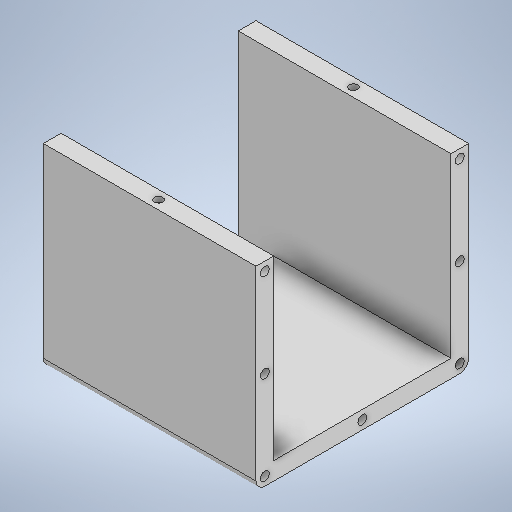
# Autodesk Inventor part: Fuselage_Body_Piece
Saved by Autodesk Inventor 2025.1 (Build 291241020, 241B)
## iProperties
Created: 2025-02-15
Part Number: Fuselage_Body_Piece
Material: Generic
Document SubType Name: Modeling
Designer: smyth
Density: 1 g/cm^3
Appearance: Default
Author: smyth
Autodesk Inventor part; units mm, degrees
ref_plane "YZ Plane" through (0, 0, 0) normal (1, 0, 0) x (0, 1, 0)
ref_plane "XZ Plane" through (0, 0, 0) normal (0, 1, 0) x (-1, 0, 0)
ref_plane "XY Plane" through (0, 0, 0) normal (0, 0, 1) x (1, 0, 0)
sketch "Sketch1" plane through (0, 0, 0) normal (0, 1, 0) x (-1, 0, 0)
  point P0 (0, 0)
sketch "Sketch2" plane through (0, 0, 0) normal (0, 1, 0) x (-1, 0, 0)
  line L0 (-76.2, 76.2) -> (76.2, 76.2)
  line L1 (76.2, 76.2) -> (76.2, -76.2)
  line L2 (76.2, -76.2) -> (-76.2, -76.2)
  line L3 (-76.2, -76.2) -> (-76.2, 76.2)
  line L4 (-76.2, 76.2) -> (76.2, -76.2) construction
  line L5 (76.2, 76.2) -> (-76.2, -76.2) construction
  point P0 (0, 0)
  dimension "d0" = 152.4
  dimension "d1" = 152.4
  constraints: 12 end point, 2 midpoint, 2 parallel, 1 horizontal, 1 perpendicular
  measures "d0" distance of L1.end L2.end
  measures "d1" distance of L0.end L1.end
extrude "Extrusion1" add sketch "Sketch2" along normal blind 12.7
sketch "Sketch3" plane through (0, 12.7, 0) normal (0, 1, 0) x (1, 0, 0)
  line L0 (76.2, 76.2) -> (-76.2, 76.2) projected
  line L1 (76.2, -76.2) -> (76.2, 76.2) projected
  line L2 (-76.2, 76.2) -> (76.2, 76.2)
  line L3 (76.2, 76.2) -> (76.2, 63.5)
  line L4 (76.2, 63.5) -> (-76.2, 63.5)
  line L5 (-76.2, 63.5) -> (-76.2, 76.2)
  line L6 (-76.2, -76.2) -> (76.2, -76.2)
  line L7 (76.2, -76.2) -> (76.2, -63.5)
  line L8 (76.2, -63.5) -> (-76.2, -63.5)
  line L9 (-76.2, -63.5) -> (-76.2, -76.2)
  point P0 (0, 0)
  point P1 (76.2, -76.2)
  dimension "d4" = 12.7
  dimension "d5" = 12.7
  dimension "d15" = 152.4
  constraints: 16 end point, 4 parallel, 2 horizontal, 2 perpendicular, 2 point on line
  measures "d4" distance between parallel lines of L4 L0
  measures "d5" distance between parallel lines of L8 L6
  measures "d15" distance of L6.start L6.end
extrude "Extrusion2" add sketch "Sketch3" along normal blind 127
fillet "Fillet1" radius 6.35 2 edges at (0, 0, 76.2) (0, 0, -76.2)
sketch "Sketch4" plane through (76.2, 12.7, -63.5) normal (1, 0, 0) x (0, 0, -1)
  circle A0 centre (-133.35, 120.65) radius 3.175
  circle A1 centre (-133.35, -6.35) radius 3.175
  circle A2 centre (-133.35, 57.15) radius 3.175
  circle A3 centre (6.35, 120.65) radius 3.175
  circle A4 centre (6.35, -6.35) radius 3.175
  circle A5 centre (6.35, 57.15) radius 3.175
  circle A6 centre (-63.5, -6.35) radius 3.175
  point P0 (-63.5, -12.7)
  dimension "d9" = 127
  constraints: 7 centre point
  measures "d9" distance of A1.centre A0.centre
extrude "Extrusion3" cut sketch "Sketch4" against normal blind 12.7
sketch "Sketch5" plane through (-76.2, 12.7, 63.5) normal (-1, 0, 0) x (0, 0, 1)
  circle A0 centre (-133.35, 120.65) radius 3.175 projected
  circle A1 centre (-133.35, 120.65) radius 3.175
  circle A2 centre (-133.35, 57.15) radius 3.175 projected
  circle A3 centre (-133.35, 57.15) radius 3.175
  circle A4 centre (-133.35, -6.35) radius 3.175 projected
  circle A5 centre (-133.35, -6.35) radius 3.175
  circle A6 centre (-63.5, -6.35) radius 3.175 projected
  circle A7 centre (-63.5, -6.35) radius 3.175
  circle A8 centre (6.35, -6.35) radius 3.175 projected
  circle A9 centre (6.35, -6.35) radius 3.175
  circle A10 centre (6.35, 57.15) radius 3.175 projected
  circle A11 centre (6.35, 57.15) radius 3.175
  circle A12 centre (6.35, 120.65) radius 3.175 projected
  circle A13 centre (6.35, 120.65) radius 3.175
  line L0 (6.35, -12.7) -> (-133.35, -12.7) projected
  point P0 (-63.5, -12.7)
  dimension "d20" = 69.85
  constraints: 7 centre point, 7 coincident
  measures "d20" distance from line of L0 A11.centre
sketch "Sketch6" plane through (0, 139.7, 0) normal (0, 1, 0) x (1, 0, 0)
  line L0 (76.2, 69.85) -> (-76.2, 69.85) projected
  circle A0 centre (0, 69.85) radius 3
  line L1 (-76.2, -69.85) -> (76.2, -69.85) projected
  circle A1 centre (0, -69.85) radius 3
  point P0 (0, 0)
  dimension "d16" = 6
  dimension "d17" = 6
  constraints: 2 centre point, 2 midpoint
  measures "d16" diameter of A0
  measures "d17" diameter of A1
extrude "Extrusion5" cut sketch "Sketch6" against normal blind 4
extrude "Extrusion6" cut sketch "Sketch5" against normal blind 12.7
body "Solid1"
